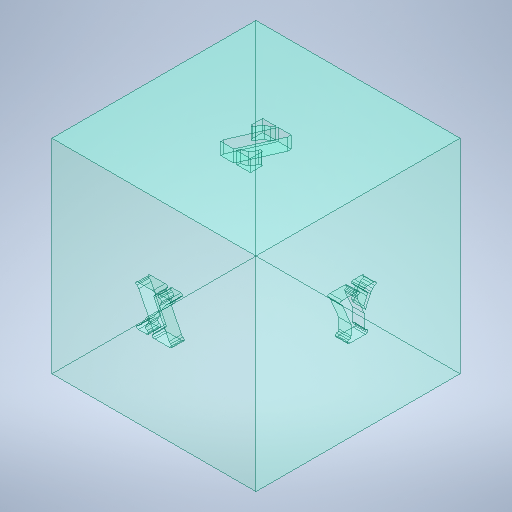
# Autodesk Inventor part: Cubo_0001_001
Saved by Autodesk Inventor 2025.2 (Build 292293000, 293)
## iProperties
Created: 2025-03-19
Part Number: Cubo_0001_001
Material: Titânio
Document SubType Name: Modeling
Designer: lucas
Density: 4.51 g/cm^3
Appearance: Borracha - Preta
Author: lucas
## iProperties of the stored document Cubo_0001_001_3DPrint.ipt
Created: 2025-03-19
Part Number: Cubo_0001_001_3DPrint
Material: Genérico
Document SubType Name: Modeling
Designer: lucas
Density: 1 g/cm^3
Appearance: Padrão
Author: lucas
Autodesk Inventor part; units mm, degrees
ref_plane "YZ Plane" through (0, 0, 0) normal (1, 0, 0) x (0, 1, 0)
ref_plane "XZ Plane" through (0, 0, 0) normal (0, 1, 0) x (-1, 0, 0)
ref_plane "XY Plane" through (0, 0, 0) normal (0, 0, 1) x (1, 0, 0)
sketch "Esboço1" plane through (0, 0, 0) normal (0, 0, 1) x (1, 0, 0)
  line L0 (-25, 25) -> (25, 25)
  line L1 (25, 25) -> (25, -25)
  line L2 (25, -25) -> (-25, -25)
  line L3 (-25, -25) -> (-25, 25)
  line L4 (-25, 25) -> (25, -25) construction
  line L5 (25, 25) -> (-25, -25) construction
  point P0 (0, 0)
  point P1 (0, 0)
  dimension "d0" = 50
  constraints: 12 end point, 2 midpoint, 2 parallel, 2 perpendicular, 1 coincident, 1 horizontal
  measures "d0" distance of L0.start L0.end
extrude "Extrusão1" add sketch "Esboço1" along normal mid plane 50
sketch "Esboço2" plane through (0, 0, 25) normal (0, 0, 1) x (1, 0, 0)
  line L0 (-4.5616, 5) -> (4.5616, 5) construction
  line L1 (4.5616, 5) -> (4.5616, -5) construction
  line L2 (4.5616, -5) -> (-4.5616, -5) construction
  line L3 (-4.5616, -5) -> (-4.5616, 5) construction
  line L4 (-4.5616, 0) -> (4.5616, 0) construction
  line L5 (0.0304, 3.7153) -> (3.7196, -3.776)
  spline S0 degree 2 poles (3.7196, -3.776) (3.8498, -4.0365) (4.0755, -4.1493) knots 0 0 0 1 1 1
  spline S1 degree 2 poles (4.0755, -4.1493) (4.2752, -4.2535) (4.4141, -4.4271) (4.4141, -4.5833) knots 0 0 0 1 2 2 2
  spline S2 degree 2 poles (4.4141, -4.5833) (4.4141, -4.783) (4.2665, -4.8958) knots 0 0 0 1 1 1
  spline S3 degree 2 poles (4.2665, -4.8958) (4.145, -5) (3.737, -5) knots 0 0 0 1 1 1
  line L6 (3.737, -5) -> (0.2995, -5)
  spline S4 degree 2 poles (0.2995, -5) (-0.0911, -5) (-0.2127, -4.9479) knots 0 0 0 1 1 1
  spline S5 degree 2 poles (-0.2127, -4.9479) (-0.4644, -4.8351) (-0.4644, -4.5747) knots 0 0 0 1 1 1
  spline S6 degree 2 poles (-0.4644, -4.5747) (-0.4644, -4.4792) (-0.3602, -4.3403) (-0.2214, -4.2361) knots 0 0 0 1 2 2 2
  spline S7 degree 2 poles (-0.2214, -4.2361) (0.0217, -4.0538) (0.013, -3.8976) knots 0 0 0 1 1 1
  spline S8 degree 2 poles (0.013, -3.8976) (0.0043, -3.776) (-0.1172, -3.5243) knots 0 0 0 1 1 1
  line L7 (-0.1172, -3.5243) -> (-3.7109, 3.7153)
  spline S9 degree 2 poles (-3.7109, 3.7153) (-3.7977, 3.8976) (-4.0061, 4.1146) (-4.171, 4.2014) knots 0 0 0 1 2 2 2
  spline S10 degree 2 poles (-4.171, 4.2014) (-4.3186, 4.2708) (-4.4314, 4.4531) (-4.4314, 4.6007) knots 0 0 0 1 2 2 2
  spline S11 degree 2 poles (-4.4314, 4.6007) (-4.4314, 4.8264) (-4.1189, 5) (-3.7109, 5) knots 0 0 0 1 2 2 2
  line L8 (-3.7109, 5) -> (-0.2995, 5)
  spline S12 degree 2 poles (-0.2995, 5) (0.0738, 5) (0.4036, 4.809) (0.4036, 4.6007) knots 0 0 0 1 2 2 2
  spline S13 degree 2 poles (0.4036, 4.6007) (0.4036, 4.3837) (0.1606, 4.2274) knots 0 0 0 1 1 1
  spline S14 degree 2 poles (0.1606, 4.2274) (0.0477, 4.1406) (-0.0304, 4.0365) (-0.0304, 3.941) knots 0 0 0 1 2 2 2
  spline S15 degree 2 poles (-0.0304, 3.941) (-0.0304, 3.8368) (0.0304, 3.7153) knots 0 0 0 1 1 1
  line L9 (-1.7752, -1.4236) -> (-1.3759, -2.2569)
  line L10 (-1.3759, -2.2569) -> (-1.8273, -3.0035)
  spline S16 degree 2 poles (-1.8273, -3.0035) (-2.079, -3.4115) (-2.079, -3.6545) knots 0 0 0 1 1 1
  spline S17 degree 2 poles (-2.079, -3.6545) (-2.079, -4.0017) (-1.6884, -4.1667) knots 0 0 0 1 1 1
  spline S18 degree 2 poles (-1.6884, -4.1667) (-1.4627, -4.2535) (-1.3064, -4.4271) (-1.3064, -4.5833) knots 0 0 0 1 2 2 2
  spline S19 degree 2 poles (-1.3064, -4.5833) (-1.3064, -4.7917) (-1.48, -4.9219) knots 0 0 0 1 1 1
  spline S20 degree 2 poles (-1.48, -4.9219) (-1.5495, -4.974) (-1.7057, -5) (-1.9314, -5) knots 0 0 0 1 2 2 2
  line L11 (-1.9314, -5) -> (-3.8238, -5)
  spline S21 degree 2 poles (-3.8238, -5) (-4.0582, -5) (-4.3273, -4.8003) (-4.3273, -4.6267) knots 0 0 0 1 2 2 2
  spline S22 degree 2 poles (-4.3273, -4.6267) (-4.3273, -4.4878) (-4.1623, -4.3056) (-3.9453, -4.2274) knots 0 0 0 1 2 2 2
  spline S23 degree 2 poles (-3.9453, -4.2274) (-3.3984, -4.0104) (-3.0946, -3.5243) knots 0 0 0 1 1 1
  line L12 (-3.0946, -3.5243) -> (-1.7752, -1.4236)
  line L13 (1.6797, 1.684) -> (1.2717, 2.5)
  line L14 (1.2717, 2.5) -> (1.6797, 3.1944)
  spline S24 degree 2 poles (1.6797, 3.1944) (1.8186, 3.4375) (1.8186, 3.6111) knots 0 0 0 1 1 1
  spline S25 degree 2 poles (1.8186, 3.6111) (1.8186, 3.776) (1.6189, 4.0799) (1.4627, 4.158) knots 0 0 0 1 2 2 2
  line L15 (1.4627, 4.158) -> (1.2023, 4.2708)
  spline S26 degree 2 poles (1.2023, 4.2708) (1.1328, 4.3142) (1.02, 4.5139) (1.02, 4.6181) knots 0 0 0 1 2 2 2
  spline S27 degree 2 poles (1.02, 4.6181) (1.02, 4.7917) (1.2717, 5) (1.4714, 5) knots 0 0 0 1 2 2 2
  line L16 (1.4714, 5) -> (3.5894, 5)
  spline S28 degree 2 poles (3.5894, 5) (3.7977, 5) (4.0668, 4.8177) (4.0668, 4.6701) knots 0 0 0 1 2 2 2
  spline S29 degree 2 poles (4.0668, 4.6701) (4.0668, 4.4965) (3.9366, 4.3663) knots 0 0 0 1 1 1
  spline S30 degree 2 poles (3.9366, 4.3663) (3.8845, 4.3142) (3.6241, 4.1753) knots 0 0 0 1 1 1
  spline S31 degree 2 poles (3.6241, 4.1753) (3.1033, 3.8889) (2.7648, 3.3507) knots 0 0 0 1 1 1
  line L17 (2.7648, 3.3507) -> (1.6797, 1.684)
  point P0 (0, 0)
  point P1 (0, 0)
  dimension "d3" = 9.1233
  dimension "d4" = 10
  constraints: 3 midpoint, 2 end point, 1 coincident, 1 horizontal, 2 other
  measures "d3" distance of L0.start L0.end
  measures "d4" distance of L2.end L0.start
extrude "Extrusão2" cut sketch "Esboço2" against normal blind 3
sketch "Esboço3" plane through (25, -25, 25) normal (1, 0, 0) x (0, 0, -1)
  line L0 (20.5208, 30) -> (29.4792, 30) construction
  line L1 (29.4792, 30) -> (29.4792, 20) construction
  line L2 (29.4792, 20) -> (20.5208, 20) construction
  line L3 (20.5208, 20) -> (20.5208, 30) construction
  line L4 (20.5208, 25) -> (29.4792, 25) construction
  line L5 (26.5365, 24.5833) -> (26.5365, 21.3889)
  spline S0 degree 2 poles (26.5365, 21.3889) (26.5365, 21.1024) (26.6493, 20.9809) knots 0 0 0 1 1 1
  spline S1 degree 2 poles (26.6493, 20.9809) (26.7014, 20.9115) (26.8056, 20.8681) (27.092, 20.7986) knots 0 0 0 1 2 2 2
  spline S2 degree 2 poles (27.092, 20.7986) (27.4479, 20.7205) (27.4479, 20.3993) knots 0 0 0 1 1 1
  spline S3 degree 2 poles (27.4479, 20.3993) (27.4479, 20.1823) (27.2483, 20.0694) knots 0 0 0 1 1 1
  spline S4 degree 2 poles (27.2483, 20.0694) (27.1354, 20) (26.7969, 20) knots 0 0 0 1 1 1
  line L6 (26.7969, 20) -> (26.5451, 20)
  line L7 (26.5451, 20) -> (23.2726, 20)
  line L8 (23.2726, 20) -> (23.0295, 20)
  spline S5 degree 2 poles (23.0295, 20) (22.6997, 20) (22.5694, 20.0868) knots 0 0 0 1 1 1
  spline S6 degree 2 poles (22.5694, 20.0868) (22.3785, 20.2083) (22.3785, 20.3993) knots 0 0 0 1 1 1
  spline S7 degree 2 poles (22.3785, 20.3993) (22.3785, 20.7205) (22.7344, 20.7986) knots 0 0 0 1 1 1
  spline S8 degree 2 poles (22.7344, 20.7986) (23.0208, 20.8681) (23.1163, 20.9115) (23.1684, 20.9809) knots 0 0 0 1 2 2 2
  spline S9 degree 2 poles (23.1684, 20.9809) (23.2813, 21.1024) (23.2813, 21.3889) knots 0 0 0 1 1 1
  line L9 (23.2813, 21.3889) -> (23.2813, 23.8628)
  line L10 (23.2813, 23.8628) -> (21.2066, 28.8108)
  spline S10 degree 2 poles (21.2066, 28.8108) (21.0938, 29.0885) (20.8767, 29.2188) knots 0 0 0 1 1 1
  spline S11 degree 2 poles (20.8767, 29.2188) (20.6858, 29.3403) (20.5729, 29.4878) (20.5729, 29.6181) knots 0 0 0 1 2 2 2
  spline S12 degree 2 poles (20.5729, 29.6181) (20.5729, 30) (21.1285, 30) knots 0 0 0 1 1 1
  line L11 (21.1285, 30) -> (24.7222, 30)
  spline S13 degree 2 poles (24.7222, 30) (25, 30) (25.1128, 29.9306) knots 0 0 0 1 1 1
  spline S14 degree 2 poles (25.1128, 29.9306) (25.2951, 29.8177) (25.2951, 29.6267) knots 0 0 0 1 1 1
  spline S15 degree 2 poles (25.2951, 29.6267) (25.2951, 29.3924) (25.0868, 29.2622) knots 0 0 0 1 1 1
  line L12 (25.0868, 29.2622) -> (24.8698, 29.1319)
  spline S16 degree 2 poles (24.8698, 29.1319) (24.7483, 29.0451) (24.7483, 28.8889) knots 0 0 0 1 1 1
  spline S17 degree 2 poles (24.7483, 28.8889) (24.7483, 28.7066) (24.8264, 28.5243) knots 0 0 0 1 1 1
  line L13 (24.8264, 28.5243) -> (26.5365, 24.5833)
  line L14 (26.8229, 25.2778) -> (26.4063, 26.2413)
  line L15 (26.4063, 26.2413) -> (27.1788, 27.9601)
  spline S18 degree 2 poles (27.1788, 27.9601) (27.2743, 28.1858) (27.2743, 28.559) knots 0 0 0 1 1 1
  spline S19 degree 2 poles (27.2743, 28.559) (27.2743, 28.9844) (26.8056, 29.1753) knots 0 0 0 1 1 1
  spline S20 degree 2 poles (26.8056, 29.1753) (26.5538, 29.2708) (26.3976, 29.4271) (26.3976, 29.592) knots 0 0 0 1 2 2 2
  spline S21 degree 2 poles (26.3976, 29.592) (26.3976, 29.7917) (26.5278, 29.8872) knots 0 0 0 1 1 1
  spline S22 degree 2 poles (26.5278, 29.8872) (26.6146, 29.9566) (26.8316, 30) (27.1094, 30) knots 0 0 0 1 2 2 2
  line L16 (27.1094, 30) -> (28.9149, 30)
  spline S23 degree 2 poles (28.9149, 30) (29.4271, 30) (29.4271, 29.592) knots 0 0 0 1 1 1
  spline S24 degree 2 poles (29.4271, 29.592) (29.4271, 29.4444) (29.2882, 29.2795) (29.0885, 29.1927) knots 0 0 0 1 2 2 2
  spline S25 degree 2 poles (29.0885, 29.1927) (28.7326, 29.0365) (28.5764, 28.8715) knots 0 0 0 1 1 1
  spline S26 degree 2 poles (28.5764, 28.8715) (28.3594, 28.6372) (28.2118, 28.3333) knots 0 0 0 1 1 1
  line L17 (28.2118, 28.3333) -> (28.0469, 27.9601)
  line L18 (28.0469, 27.9601) -> (26.8229, 25.2778)
  point P0 (25, 25)
  point P1 (25, 25)
  dimension "d7" = 8.9583
  dimension "d8" = 10
  constraints: 3 midpoint, 2 end point, 1 coincident, 1 horizontal, 2 other
  measures "d7" distance of L0.start L0.end
  measures "d8" distance of L2.end L0.start
extrude "Extrusão3" cut sketch "Esboço3" against normal blind 3
sketch "Esboço4" plane through (-25, 25, 25) normal (0, 1, 0) x (1, 0, 0)
  line L0 (21.072, 30) -> (28.928, 30) construction
  line L1 (28.928, 30) -> (28.928, 20) construction
  line L2 (28.928, 20) -> (21.072, 20) construction
  line L3 (21.072, 20) -> (21.072, 30) construction
  line L4 (21.072, 25) -> (28.928, 25) construction
  line L5 (28.6241, 30) -> (28.6241, 29.158)
  line L6 (28.6241, 29.158) -> (24.579, 20)
  line L7 (24.579, 20) -> (21.3759, 20)
  line L8 (21.3759, 20) -> (21.3759, 20.7292)
  line L9 (21.3759, 20.7292) -> (25.4384, 30)
  line L10 (25.4384, 30) -> (28.6241, 30)
  line L11 (28.6241, 20) -> (25.1953, 20)
  line L12 (25.1953, 20) -> (25.5252, 20.7292)
  spline S0 degree 2 poles (25.5252, 20.7292) (26.428, 20.9462) (26.8273, 21.224) knots 0 0 0 1 1 1
  spline S1 degree 2 poles (26.8273, 21.224) (27.1745, 21.467) (27.5998, 22.092) (27.8342, 22.7257) knots 0 0 0 1 2 2 2
  spline S2 degree 2 poles (27.8342, 22.7257) (27.921, 22.9601) (28.0859, 23.125) (28.2335, 23.125) knots 0 0 0 1 2 2 2
  spline S3 degree 2 poles (28.2335, 23.125) (28.4245, 23.125) (28.6241, 22.8646) (28.6241, 22.6128) knots 0 0 0 1 2 2 2
  line L13 (28.6241, 22.6128) -> (28.6241, 20)
  line L14 (21.6189, 30) -> (24.796, 30)
  line L15 (24.796, 30) -> (24.4314, 29.1667)
  spline S4 degree 2 poles (24.4314, 29.1667) (23.8064, 29.0799) (23.2856, 28.7066) knots 0 0 0 1 1 1
  spline S5 degree 2 poles (23.2856, 28.7066) (22.6259, 28.2465) (22.3915, 27.3785) knots 0 0 0 1 1 1
  spline S6 degree 2 poles (22.3915, 27.3785) (22.3307, 27.1528) (22.1571, 26.9792) (21.9922, 26.9792) knots 0 0 0 1 2 2 2
  spline S7 degree 2 poles (21.9922, 26.9792) (21.6189, 26.9792) (21.6189, 27.4045) knots 0 0 0 1 1 1
  line L16 (21.6189, 27.4045) -> (21.6189, 30)
  point P0 (25, 25)
  point P1 (25, 25)
  dimension "d11" = 7.8559
  dimension "d12" = 10
  constraints: 3 midpoint, 2 end point, 1 coincident, 2 other
  measures "d11" distance of L0.start L0.end
  measures "d12" distance of L2.end L0.start
extrude "Extrusão4" cut sketch "Esboço4" against normal blind 3
equation "\"d1\" = d0"
